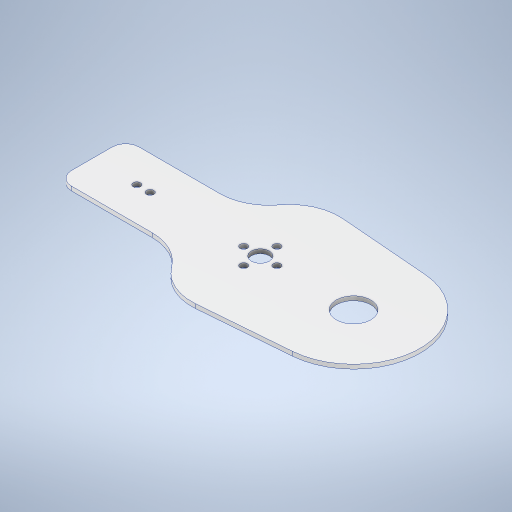
# Autodesk Inventor part: Wrist Side Brase
Saved by Autodesk Inventor 2023 (Build 270158030, 158C)
## iProperties
Created: 2022-09-21
Part Number: Wrist Side Brase
Material: Aluminum 6061
Document SubType Name: Modeling
Designer: caden
Density: 2.7 g/cm^3
Appearance: Aluminum - Flat
Mass: 158.416 g
Surface Area: 396.255 cm^2
Volume: 58.6727 cm^3
Author: caden
Autodesk Inventor part; units mm, degrees
ref_plane "YZ Plane" through (0, 0, 0) normal (1, 0, 0) x (0, 1, 0)
ref_plane "XZ Plane" through (0, 0, 0) normal (0, 1, 0) x (-1, 0, 0)
ref_plane "XY Plane" through (0, 0, 0) normal (0, 0, 1) x (1, 0, 0)
sketch "Sketch1" plane through (0, 0, 0) normal (0, 1, 0) x (-1, 0, 0)
  arc A0 (-4.0306, 49.8373) -> (-4.0306, -49.8373) centre (0, 0) ccw
  arc A1 (155.977, -62.778) -> (196.5, -25.4) centre (159, -25.4) ccw
  arc A2 (196.5, 25.4) -> (155.977, 62.778) centre (159, 25.4) ccw
  line L0 (155.977, -62.778) -> (-4.0306, -49.8373)
  line L1 (155.977, 62.778) -> (-4.0306, 49.8373)
  line L2 (196.5, -25.4) -> (196.5, 25.4)
  line L3 (0, 0) -> (1115.1702, 0)
  dimension "d0" = 75
  dimension "d1" = 159
  dimension "d2" = 50.8
  dimension "d3" = 50
  constraints: 8 end point, 6 point on circle, 6 tangent, 3 centre point, 1 coincident, 1 equal radius, 1 horizontal, 1 symmetric about line, 1 vertical
  measures "d0" diameter of A1
  measures "d1" horizontal distance of point (0, 0) A1.centre
  measures "d2" distance of A1.centre A2.centre
  measures "d3" radius of A0
extrude "Main" add sketch "Sketch1" along normal blind 3.175
sketch "Sketch2" plane through (0, 3.175, 0) normal (0, 1, 0) x (1, 0, 0)
  circle A0 centre (0, 0) radius 13
  circle A1 centre (-70, 0) radius 6.75
  arc A2 (-196.5, -25.4) -> (-155.977, -62.778) centre (-159, -25.4) ccw projected
  arc A3 (-155.977, 62.778) -> (-196.5, 25.4) centre (-159, 25.4) ccw projected
  line L0 (0, 0) -> (-245.2379, 0)
  dimension "d6" = 13.5
  dimension "d40" = 26
  dimension "d41" = 70
  constraints: 2 centre point, 2 end point, 1 coincident, 1 horizontal, 1 point on line
  measures "d6" diameter of A1
  measures "d40" diameter of A0
  measures "d41" distance of point (0, 0) A1.centre
extrude "Axis Holes" cut sketch "Sketch2" against normal through all
sketch "Sketch5" plane through (0, 3.175, 0) normal (0, 1, 0) x (1, 0, 0)
  line L0 (-145.7, 0) -> (-145.7, 35.4875) construction
  line L1 (-196.5, 25.4) -> (-196.5, -25.4) construction
  circle A0 centre (-152.7, 0) radius 2.75
  circle A1 centre (-162.7, 0) radius 2.75
  point P0 (0, 0)
  dimension "d43" = 50.8
  dimension "d44" = 7
  dimension "d45" = 10
  dimension "d46" = 5.5
  constraints: 2 centre point, 2 end point, 1 equal radius, 1 vertical
  measures "d43" distance between parallel lines of L0 L1
  measures "d44" distance from line of L0 A0.centre
  measures "d45" distance of A1.centre A0.centre
  measures "d46" diameter of A1
extrude "Extrusion6" cut sketch "Sketch5" against normal through all
sketch "Sketch6" plane through (0, 3.175, 0) normal (0, 1, 0) x (1, 0, 0)
  line L0 (-196.5, 25.4) -> (-196.5, -25.4) projected
  line L1 (-196.5, 25.4) -> (-106.5, 25.4)
  line L2 (-106.5, -25.4) -> (-196.5, -25.4)
  line L3 (-196.5, -25.4) -> (-196.5, 25.4)
  line L4 (0, 0) -> (-211.532, 0)
  line L5 (-106.5, -25.4) -> (-84.6567, -57.0099)
  line L6 (-106.5, 25.4) -> (-84.6567, 57.0099)
  line L7 (4.0306, 49.8373) -> (-155.977, 62.778) projected
  arc A0 (-155.977, 62.778) -> (-196.5, 25.4) centre (-159, 25.4) ccw projected
  arc A1 (-155.977, 62.778) -> (-196.5, 25.4) centre (-159, 25.4) ccw
  line L8 (-155.977, -62.778) -> (4.0306, -49.8373) projected
  arc A2 (-196.5, -25.4) -> (-155.977, -62.778) centre (-159, -25.4) ccw
  line L9 (-155.977, -62.778) -> (-84.6567, -57.0099)
  line L10 (-84.6567, 57.0099) -> (-155.977, 62.778)
  line L11 (4.0306, 49.8373) -> (-155.977, 62.778) projected
  point P0 (-66.0008, 55.5011)
  point P1 (-69.732, 55.8029)
  point P2 (-155.977, 62.778)
  dimension "d49" = 50.8
  dimension "d50" = 90
  constraints: 16 end point, 4 point on circle, 3 point on line, 2 centre point, 2 horizontal, 2 symmetric about line, 1 collinear, 1 parallel, 1 vertical
  measures "d49" distance of L1.end L2.start
  measures "d50" distance of L2.start L2.end
extrude "Extrusion7" cut sketch "Sketch6" against normal through all
fillet "Fillet1" radius 36.925 4 edges at (-106.5, 1.5875, -25.4) (-84.6567, 1.5875, -57.0099) (-84.6567, 1.5875, 57.0099) (-106.5, 1.5875, 25.4)
fillet "Fillet2" radius 10 2 edges at (-196.5, 1.5875, -25.4) (-196.5, 1.5875, 25.4)
sketch "Sketch7" plane through (0, 3.175, 0) normal (0, 1, 0) x (1, 0, 0)
  circle A0 centre (-70, 0) radius 6.75 construction
  circle A1 centre (-70, 0) radius 12.5 construction
  circle A2 centre (-70, 12.5) radius 2.75
  circle A3 centre (-82.5, 0) radius 2.75
  circle A4 centre (-70, -12.5) radius 2.75
  circle A5 centre (-57.5, 0) radius 2.75
  point P0 (0, 0)
  dimension "d63" = 25
  dimension "d58" = 5.5
  dimension "d61" = 360
  constraints: 4 centre point, 1 coincident, 1 vertical alignment, 11 other
  measures "d58" diameter of A2
extrude "Extrusion8" cut sketch "Sketch7" against normal blind 10
body "Solid1"
